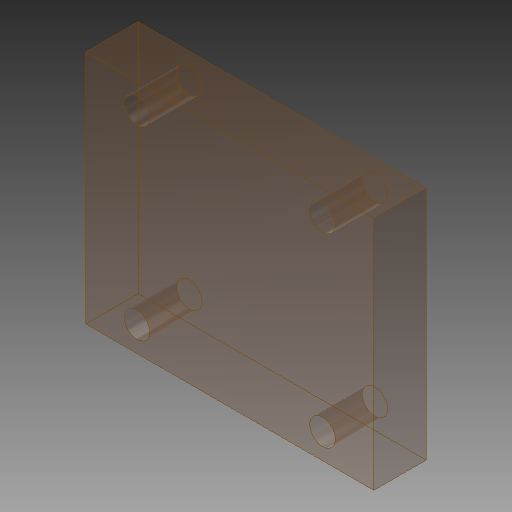
# Autodesk Inventor part: polycarb_back
Saved by Autodesk Inventor 2018.1 (Build 221171000, 171)
## iProperties
Created: 2017-08-10
Part Number: polycarb_back
Material: Polycarbonate, Smoke
Document SubType Name: Modeling
Designer: Kai
Density: 1.2 g/cm^3
Appearance: Polycarbonate - Smoked
Author: Kai
Autodesk Inventor part; units mm, degrees
ref_plane "YZ Plane" through (0, 0, 0) normal (1, 0, 0) x (0, 1, 0)
ref_plane "XZ Plane" through (0, 0, 0) normal (0, 1, 0) x (-1, 0, 0)
ref_plane "XY Plane" through (0, 0, 0) normal (0, 0, 1) x (1, 0, 0)
sketch "Sketch1" plane through (0, 0, 0) normal (0, 0, 1) x (1, 0, 0)
  line L0 (0, 0) -> (57.15, 0)
  line L1 (57.15, 0) -> (57.15, 57.15)
  line L2 (57.15, 57.15) -> (0, 57.15)
  line L3 (0, 57.15) -> (0, 0)
  line L4 (0, 57.15) -> (57.15, 0) construction
  circle A0 centre (28.575, 28.575) radius 31.825 construction
  line L5 (0, 0) -> (57.15, 57.15) construction
  circle A1 centre (6.0713, 51.0787) radius 3.1
  circle A2 centre (6.0713, 6.0713) radius 3.1
  circle A3 centre (51.0787, 6.0713) radius 3.1
  circle A4 centre (51.0787, 51.0787) radius 3.1
  dimension "d2" = 63.65
  dimension "d0" = 57.15
  dimension "d1" = 57.15
  dimension "d3" = 6.2
  dimension "d6" = 360
  constraints: 12 end point, 4 centre point, 2 parallel, 1 horizontal, 1 midpoint, 1 perpendicular, 1 point on line, 12 other
  measures "d0" distance of L2.end L1.end
  measures "d1" distance of L1.end L0.end
  measures "d3" diameter of A1
extrude "Extrusion1" add sketch "Sketch1" along normal blind 12.7
sketch "Sketch2" plane through (0, 0, 12.7) normal (0, 0, 1) x (1, 0, 0)
  line L0 (0, 0) -> (-6.35, 0)
  line L1 (-6.35, 0) -> (-6.35, 57.15)
  line L2 (-6.35, 57.15) -> (0, 57.15)
  line L3 (0, 57.15) -> (0, 0)
  line L4 (57.15, 0) -> (57.15, 57.15) projected
  line L5 (57.15, 57.15) -> (63.5, 57.15)
  line L6 (63.5, 57.15) -> (63.5, 0)
  line L7 (63.5, 0) -> (57.15, 0)
  line L8 (57.15, 0) -> (57.15, 57.15)
  dimension "d10" = 6.35
  dimension "d11" = 6.35
  constraints: 16 end point, 4 parallel, 2 horizontal, 2 perpendicular, 1 point on line
  measures "d10" distance of L1.end L2.end
  measures "d11" distance of L6.end L7.end
extrude "Extrusion2" add sketch "Sketch2" against normal up to surface (12.7 mm away)
body "Solid1"
